Sholder Part 2_v1 (Autodesk Fusion 360 design; units mm, degrees)
Autodesk Fusion 360 part; units mm, degrees
sketch "Sketch1" plane through (0, 0, 0) normal (0, 0, 1) x (1, 0, 0)
  circle A0 centre (0, 0) radius 42.75
  circle A1 centre (0, 0) radius 39.5
  line L0 (0, 0) -> (0, -100) construction
  line L1 (100, -105) -> (-100, -105)
  line L2 (-100, -105) -> (-100, -95)
  line L3 (100, -95) -> (100, -105)
  line L4 (100, -105) -> (-100, -95) construction
  line L5 (-100, -105) -> (100, -95) construction
  circle A2 centre (0, 0) radius 52.5
  line L6 (-52.5, 0) -> (-52.5, -57.5)
  line L7 (52.5, 0) -> (52.5, -57.5)
  line L8 (-100, -95) -> (-90, -95)
  line L9 (90, -95) -> (100, -95)
  arc A3 (-90, -95) -> (-52.5, -57.5) centre (-90, -57.5) ccw
  arc A4 (52.5, -57.5) -> (90, -95) centre (90, -57.5) ccw
  point P0 (0, -100)
  dimension "d1" = 85.5
  dimension "d5" = 79
  dimension "d7" = 100
  dimension "d8" = 200
  dimension "d9" = 10
  dimension "d10" = 105
  dimension "d11" = 37.5
  dimension "d12" = 10
  dimension "d13" = 37.5
  constraint coincident A0.centre A1.centre
  constraint vertical L0
  constraint horizontal L1
  constraint perpendicular L1 L2
  constraint parallel L1 L8
  constraint parallel L2 L3
  constraint coincident L4 P0
  constraint coincident L5 P0
  constraint coincident P0 L0.end
  constraint concentric A0 A2
  constraint coincident A2 L6.start
  constraint tangent A2 L6
  constraint perpendicular L6 L8
  constraint coincident A2 L7.start
  constraint tangent A2 L7
  constraint perpendicular L7 L8
  constraint collinear L8 L9
  constraint tangent L6 A3
  constraint tangent L8 A3
  constraint tangent L7 A4
  constraint tangent L9 A4
  measures "d1" diameter of A0
  measures "d5" diameter of A1
  measures "d7" distance of A0.centre P0
  measures "d8" distance of L2.end L3.start
  measures "d9" distance of L1.end L2.end
  measures "d10" diameter of A2
  measures "d11" radius of A3
  measures "d12" distance of L2.end L8.end
  measures "d13" radius of A4
extrude "Extrude1" add sketch "Sketch1" along normal blind 12 contours L1 L2 L3 A2 L6 L7 L8 L9 A3 A4 | A2
extrude "Extrude2" add sketch "Sketch1" along normal blind 2 contours A0
hole "Hole1" at (-95, -95, 6) direction (0, -1, 0) diameter 3 depth 10 tip angle 118
hole "Hole2" at (95.5037, -95, 6.5484) direction (0, -1, 0) diameter 3 depth 10 tip angle 118
equation "d1 = BearingDia + Tollerance"
equation "BearingDia = 85 mm"
equation "BearingOffset = 79 mm"
equation "Tollerance = 0.5 mm"
equation "d5 = BearingOffset"
equation "AxleHeight = 105 mm"
equation "d7 = AxleHeight - 5 mm"
equation "d10 = BearingDia + 20 mm"
